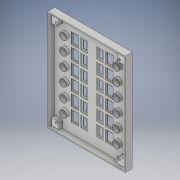
# Autodesk Inventor part: TestTapa_v2
Saved by Autodesk Inventor 2019 (Build 230136000, 136)
## iProperties
Created: 2019-05-27
Part Number: TestTapa_v2
Material: Genérico
Document SubType Name: Modeling
Designer: LuisAlonso
Density: 1 g/cm^3
Appearance: Valor por defecto
Author: LuisAlonso
Autodesk Inventor part; units mm, degrees
(part 1 of 2)
ref_plane "YZ Plane" through (0, 0, 0) normal (1, 0, 0) x (0, 1, 0)
ref_plane "XZ Plane" through (0, 0, 0) normal (0, 1, 0) x (-1, 0, 0)
ref_plane "XY Plane" through (0, 0, 0) normal (0, 0, 1) x (1, 0, 0)
sketch "Boceto1" plane through (0, 0, 0) normal (0, 0, 1) x (1, 0, 0)
  line L0 (-83, -108.2) -> (83, -108.2)
  line L1 (83, -108.2) -> (83, 108.2)
  line L2 (83, 108.2) -> (-83, 108.2)
  line L3 (-83, 108.2) -> (-83, -108.2)
  line L4 (-83, -108.2) -> (83, 108.2) construction
  line L5 (83, -108.2) -> (-83, 108.2) construction
  point P0 (0, 0)
  dimension "d0" = 166
  dimension "d1" = 216.4
  constraints: 12 end point, 2 midpoint, 2 parallel, 1 horizontal, 1 perpendicular
  measures "d0" distance of L2.end L1.end
  measures "d1" distance of L1.end L0.end
extrude "Extrusión1" add sketch "Boceto1" along normal blind 15
sketch "Boceto2" plane through (0, 0, 15) normal (0, 0, 1) x (1, 0, 0)
  line L0 (80.75, -105.95) -> (-80.75, -105.95)
  line L1 (-80.75, -105.95) -> (-80.75, 105.95)
  line L2 (80.75, 105.95) -> (-80.75, 105.95)
  line L3 (80.75, 105.95) -> (80.75, -105.95)
  line L4 (-83, 108.2) -> (83, 108.2)
  line L5 (83, 108.2) -> (83, -108.2)
  line L6 (83, -108.2) -> (-83, -108.2)
  line L7 (-83, -108.2) -> (-83, 108.2)
  point P0 (0, 0)
  constraints: 16 end point, 4 perpendicular, 2 parallel, 1 horizontal
extrude "Extrusión2" cut sketch "Boceto2" against normal blind 12 contours L0 L1 L2 L3
sketch "Boceto3" plane through (0, 0, 3) normal (0, 0, 1) x (1, 0, 0)
  line L0 (-67.5, -92.5) -> (67.5, -92.5)
  line L1 (67.5, -92.5) -> (67.5, 92.5)
  line L2 (67.5, 92.5) -> (-67.5, 92.5)
  line L3 (-67.5, 92.5) -> (-67.5, -92.5)
  line L4 (-67.5, 87.5) -> (-72.5, 87.5)
  line L5 (-62.5, 97.5) -> (-62.5, 92.5)
  line L6 (62.5, -97.5) -> (62.5, -92.5)
  line L7 (67.5, -87.5) -> (72.5, -87.5)
  line L8 (-72.5, -87.5) -> (-67.5, -87.5)
  line L9 (-62.5, -92.5) -> (-62.5, -97.5)
  line L10 (-72.5, 87.5) -> (-77.5, 87.5)
  line L11 (-77.5, 87.5) -> (-77.5, 102.5)
  line L12 (-77.5, 102.5) -> (-62.5, 102.5)
  line L13 (-62.5, 102.5) -> (-62.5, 97.5)
  line L14 (77.5, 87.5) -> (77.5, 102.5)
  line L15 (77.5, 102.5) -> (62.5, 102.5)
  line L16 (67.5, -87.5) -> (77.5, -87.5)
  line L17 (62.5, -92.5) -> (62.5, -102.5)
  line L18 (62.5, -102.5) -> (77.5, -102.5)
  line L19 (77.5, -102.5) -> (77.5, -87.5)
  line L20 (-67.5, -87.5) -> (-77.5, -87.5)
  line L21 (-77.5, -87.5) -> (-77.5, -102.5)
  line L22 (-77.5, -102.5) -> (-62.5, -102.5)
  line L23 (-62.5, -102.5) -> (-62.5, -97.5)
  line L24 (67.5, 87.5) -> (77.5, 87.5)
  line L25 (62.5, 102.5) -> (62.5, 92.5)
  arc A0 (-62.5, -92.5) -> (-67.5, -87.5) centre (-67.5, -92.5) ccw
  arc A1 (-67.5, 87.5) -> (-62.5, 92.5) centre (-67.5, 92.5) ccw
  arc A2 (62.5, 92.5) -> (67.5, 87.5) centre (67.5, 92.5) ccw
  arc A3 (67.5, -87.5) -> (62.5, -92.5) centre (67.5, -92.5) ccw
  point P0 (0, 0)
  dimension "d12" = 135
  dimension "d13" = 185
  dimension "d56" = 5
  dimension "d57" = 15
  dimension "d58" = 15
  constraints: 52 end point, 10 perpendicular, 8 point on circle, 6 point on line, 4 centre point, 4 coincident, 4 horizontal, 3 vertical, 2 midpoint, 1 collinear
  measures "d12" distance of L0.start L0.end
  measures "d13" distance of L0.end L1.end
  measures "d56" distance of L4.end L10.end
  measures "d57" distance of L10.end L11.end
  measures "d58" distance of L11.end L12.end
extrude "Extrusión3" add sketch "Boceto3" along normal blind 9 contours L3 A0 L0 | L0 L9 L23 L22 L21 L20 L8 L3 | A3 L1 L0 | L0 L1 L7 L16 L19 L18 L17 L6 | L4 L10 L11 L12 L13 L5 L2 L3 | L3 L2 A1 | A2 L2 L1 | L1 L2 L25 L15 L14 L24
sketch "Boceto4" plane through (0, 0, 0) normal (0, 0, -1) x (-1, 0, 0)
  line L0 (80.75, -105.95) -> (80.75, 105.95) projected
  line L1 (-80.75, -105.95) -> (80.75, -105.95) projected
  line L2 (-80.75, 105.95) -> (-80.75, -105.95) projected
  line L3 (80.75, 105.95) -> (-80.75, 105.95) projected
  line L4 (-67.5, -92.5) -> (-67.5, 92.5) projected
  line L5 (67.5, 92.5) -> (67.5, -92.5) projected
  line L6 (-67.5, 92.5) -> (67.5, 92.5) projected
  line L7 (67.5, -92.5) -> (-67.5, -92.5) projected
  circle A0 centre (-67.5, 92.5) radius 4.75
  circle A1 centre (67.5, 92.5) radius 4.75
  circle A2 centre (67.5, -92.5) radius 4.75
  circle A3 centre (-67.5, -92.5) radius 4.75
  point P0 (0, 0)
  dimension "d24" = 9.5
  dimension "d25" = 9.5
  dimension "d26" = 9.5
  dimension "d27" = 9.5
  constraints: 4 centre point, 4 coincident
  measures "d24" diameter of A0
  measures "d25" diameter of A1
  measures "d26" diameter of A2
  measures "d27" diameter of A3
extrude "Extrusión4" cut sketch "Boceto4" against normal blind 4.5 contours L7 A3 L4 | L4 A3 L7 | A0 L6 L4 | L4 L6 A0 | A2 L5 L7 | L7 L5 A2 | A1 L5 L6 | L6 L5 A1
sketch "Boceto7" plane through (-67.5, 92.5, 4.5) normal (0, 0, -1) x (-1, 0, 0)
  arc A0 (-0.8744, -2.2886) -> (-2.2886, -0.8744) centre (0, 0) ccw
  line L0 (0, 0) -> (4.75, 0) construction
  line L1 (-2.2886, -0.8744) -> (-3.9906, -2.5764)
  line L2 (-0.8744, -2.2886) -> (-2.5764, -3.9906)
  arc A1 (-3.9906, -2.5764) -> (-2.5764, -3.9906) centre (0, 0) ccw
  arc A2 (-132.7114, -0.8744) -> (-134.1256, -2.2886) centre (-135, 0) ccw
  line L3 (-134.1256, -2.2886) -> (-132.4236, -3.9906)
  line L4 (-132.7114, -0.8744) -> (-131.0094, -2.5764)
  arc A3 (-132.4236, -3.9906) -> (-131.0094, -2.5764) centre (-135, 0) ccw
  arc A4 (-134.1256, -182.7114) -> (-132.7114, -184.1256) centre (-135, -185) ccw
  line L5 (-132.7114, -184.1256) -> (-131.0094, -182.4236)
  line L6 (-134.1256, -182.7114) -> (-132.4236, -181.0094)
  arc A5 (-131.0094, -182.4236) -> (-132.4236, -181.0094) centre (-135, -185) ccw
  arc A6 (-2.2886, -184.1256) -> (-0.8744, -182.7114) centre (0, -185) ccw
  line L7 (-0.8744, -182.7114) -> (-2.5764, -181.0094)
  line L8 (-2.2886, -184.1256) -> (-3.9906, -182.4236)
  arc A7 (-2.5764, -181.0094) -> (-3.9906, -182.4236) centre (0, -185) ccw
  point P0 (-67.5, -92.5)
  constraints: 18 end point, 16 point on circle, 8 centre point, 1 horizontal
extrude "Extrusión7" cut sketch "Boceto7" against normal blind 10
sketch "Boceto8" plane through (0, 0, 3) normal (0, 0, 1) x (1, 0, 0)
  line L0 (80.75, -105.95) -> (-80.75, -105.95) projected
  line L1 (-62.5, -105.95) -> (-57.5, -105.95)
  line L2 (-57.5, -100.95) -> (57.5161, -100.95)
  line L3 (67.5, -87.5) -> (77.5, -87.5) projected
  line L4 (57.5161, -92.5) -> (57.5161, -100.95)
  line L5 (-57.5, -100.95) -> (-57.5, -92.5)
  line L6 (-67.5, -82.5) -> (-75.75, -82.5)
  line L7 (-77.5, 87.5) -> (-67.5, 87.5) projected
  line L8 (-62.5, 92.5) -> (-62.5, 102.5) projected
  line L9 (-80.75, 105.95) -> (80.75, 105.95) projected
  line L10 (-75.75, 82.5) -> (-67.5, 82.5)
  line L11 (-57.5, 92.5) -> (-57.5, 100.95)
  line L12 (-75.75, -82.5) -> (-75.75, 82.5)
  line L13 (-57.5, 100.95) -> (57.5161, 100.95)
  line L14 (57.5161, 100.95) -> (57.5161, 91.9319)
  line L15 (67.5, 82.5) -> (75.75, 82.5)
  line L16 (75.75, 82.5) -> (75.75, -82.5161)
  arc A0 (65.2114, -91.6256) -> (66.6256, -90.2114) centre (67.5, -92.5) ccw projected
  line L17 (67.5, -82.5161) -> (75.75, -82.5161)
  arc A1 (-66.6256, -90.2114) -> (-65.2114, -91.6256) centre (-67.5, -92.5) ccw projected
  arc A2 (-57.5, -92.5) -> (-67.5, -82.5) centre (-67.5, -92.5) ccw
  arc A3 (-65.2114, 91.6256) -> (-66.6256, 90.2114) centre (-67.5, 92.5) ccw projected
  arc A4 (-67.5, 82.5) -> (-57.5, 92.5) centre (-67.5, 92.5) ccw
  arc A5 (67.5, -82.5161) -> (57.5161, -92.5) centre (67.5, -92.5) ccw
  arc A6 (66.6256, 90.2114) -> (65.2114, 91.6256) centre (67.5, 92.5) ccw projected
  arc A7 (57.5, 92.5) -> (67.5, 82.5) centre (67.5, 92.5) ccw
  point P0 (0, 0)
  constraints: 26 end point, 9 point on circle, 4 centre point, 4 coincident, 4 horizontal, 4 perpendicular, 2 point on line, 2 vertical
sketch "Boceto9" plane through (0, 0, 3) normal (0, 0, 1) x (1, 0, 0)
  line L0 (0, 100.8776) -> (0, -101.1224)
  line L1 (0, 100.8776) -> (0, 72.0206)
  line L2 (0, 72.0206) -> (0, 43.1636)
  line L3 (0, 43.1636) -> (0, 14.3066)
  line L4 (0, 14.3066) -> (0, -14.5504)
  line L5 (0, -14.5504) -> (0, -43.4074)
  line L6 (0, -43.4074) -> (0, -72.2644)
  line L7 (0, -72.2644) -> (0, -101.1214)
  line L8 (0, 72.0206) -> (10, 72.0206)
  line L9 (10, 72.0206) -> (24, 72.0206)
  line L10 (24, 72.0206) -> (29, 72.0206)
  line L11 (29, 72.0206) -> (45, 72.0206)
  line L12 (45, 72.0206) -> (50, 72.0206)
  line L13 (50, 72.0206) -> (56.75, 72.0206)
  circle A0 centre (56.75, 72.0206) radius 6.75
  line L14 (30.5, 62.1456) -> (30.5, 81.8956)
  line L15 (30.5, 81.8956) -> (43.5, 81.8956)
  line L16 (43.5, 81.8956) -> (43.5, 62.1456)
  line L17 (43.5, 62.1456) -> (30.5, 62.1456)
  line L18 (30.5, 62.1456) -> (43.5, 81.8956) construction
  line L19 (30.5, 81.8956) -> (43.5, 62.1456) construction
  line L20 (13, 63.5206) -> (13, 80.5206)
  line L21 (13, 80.5206) -> (21, 80.5206)
  line L22 (21, 80.5206) -> (21, 63.5206)
  line L23 (21, 63.5206) -> (13, 63.5206)
  line L24 (13, 63.5206) -> (21, 80.5206) construction
  line L25 (13, 80.5206) -> (21, 63.5206) construction
  line L26 (0, 72.0206) -> (-10, 72.0206)
  line L27 (-10, 72.0206) -> (-24, 72.0206)
  line L28 (-24, 72.0206) -> (-29, 72.0206)
  line L29 (-29, 72.0206) -> (-45, 72.0206)
  line L30 (-45, 72.0206) -> (-50, 72.0206)
  line L31 (-50, 72.0206) -> (-56.75, 72.0206)
  circle A1 centre (-56.75, 72.0206) radius 6.75
  line L32 (-30.5, 62.1456) -> (-30.5, 81.8956)
  line L33 (-30.5, 81.8956) -> (-43.5, 81.8956)
  line L34 (-43.5, 81.8956) -> (-43.5, 62.1456)
  line L35 (-43.5, 62.1456) -> (-30.5, 62.1456)
  line L36 (-30.5, 62.1456) -> (-43.5, 81.8956) construction
  line L37 (-30.5, 81.8956) -> (-43.5, 62.1456) construction
  line L38 (-13, 63.5206) -> (-13, 80.5206)
  line L39 (-13, 80.5206) -> (-21, 80.5206)
  line L40 (-21, 80.5206) -> (-21, 63.5206)
  line L41 (-21, 63.5206) -> (-13, 63.5206)
  line L42 (-13, 63.5206) -> (-21, 80.5206) construction
  line L43 (-13, 80.5206) -> (-21, 63.5206) construction
  line L44 (0, 43.1636) -> (10, 43.1636)
  line L45 (10, 43.1636) -> (24, 43.1636)
  line L46 (24, 43.1636) -> (29, 43.1636)
  line L47 (29, 43.1636) -> (45, 43.1636)
  line L48 (45, 43.1636) -> (50, 43.1636)
  line L49 (50, 43.1636) -> (56.75, 43.1636)
  circle A2 centre (56.75, 43.1636) radius 6.75
  line L50 (30.5, 33.2886) -> (30.5, 53.0386)
  line L51 (30.5, 53.0386) -> (43.5, 53.0386)
  line L52 (43.5, 53.0386) -> (43.5, 33.2886)
  line L53 (43.5, 33.2886) -> (30.5, 33.2886)
  line L54 (30.5, 33.2886) -> (43.5, 53.0386) construction
  line L55 (30.5, 53.0386) -> (43.5, 33.2886) construction
  line L56 (13, 34.6636) -> (13, 51.6636)
  line L57 (13, 51.6636) -> (21, 51.6636)
  line L58 (21, 51.6636) -> (21, 34.6636)
  line L59 (21, 34.6636) -> (13, 34.6636)
  line L60 (13, 34.6636) -> (21, 51.6636) construction
  line L61 (13, 51.6636) -> (21, 34.6636) construction
  line L62 (-30.5, 33.2886) -> (-30.5, 53.0386)
  line L63 (-43.5, 33.2886) -> (-30.5, 33.2886)
  line L64 (-30.5, 33.2886) -> (-43.5, 53.0386) construction
  line L65 (-30.5, 53.0386) -> (-43.5, 33.2886) construction
  line L66 (-30.5, 53.0386) -> (-43.5, 53.0386)
  line L67 (-29, 43.1636) -> (-45, 43.1636)
  line L68 (-43.5, 53.0386) -> (-43.5, 33.2886)
  line L69 (-45, 43.1636) -> (-50, 43.1636)
  line L70 (-50, 43.1636) -> (-56.75, 43.1636)
  circle A3 centre (-56.75, 43.1636) radius 6.75
  line L71 (-21, 34.6636) -> (-13, 34.6636)
  line L72 (0, 43.1636) -> (-10, 43.1636)
  line L73 (-10, 43.1636) -> (-24, 43.1636)
  line L74 (-24, 43.1636) -> (-29, 43.1636)
  line L75 (-13, 34.6636) -> (-13, 51.6636)
  line L76 (-21, 51.6636) -> (-21, 34.6636)
  line L77 (-13, 51.6636) -> (-21, 51.6636)
  line L78 (-13, 34.6636) -> (-21, 51.6636) construction
  line L79 (-13, 51.6636) -> (-21, 34.6636) construction
  line L80 (0, 14.3066) -> (10, 14.3066)
  line L81 (10, 14.3066) -> (24, 14.3066)
  line L82 (24, 14.3066) -> (29, 14.3066)
  line L83 (29, 14.3066) -> (45, 14.3066)
  line L84 (45, 14.3066) -> (50, 14.3066)
  line L85 (50, 14.3066) -> (56.75, 14.3066)
  circle A4 centre (56.75, 14.3066) radius 6.75
  line L86 (30.5, 4.4316) -> (30.5, 24.1816)
  line L87 (30.5, 24.1816) -> (43.5, 24.1816)
  line L88 (43.5, 24.1816) -> (43.5, 4.4316)
  line L89 (43.5, 4.4316) -> (30.5, 4.4316)
  line L90 (30.5, 4.4316) -> (43.5, 24.1816) construction
  line L91 (30.5, 24.1816) -> (43.5, 4.4316) construction
  line L92 (13, 5.8066) -> (13, 22.8066)
  line L93 (13, 22.8066) -> (21, 22.8066)
  line L94 (21, 22.8066) -> (21, 5.8066)
  line L95 (21, 5.8066) -> (13, 5.8066)
  line L96 (13, 5.8066) -> (21, 22.8066) construction
  line L97 (13, 22.8066) -> (21, 5.8066) construction
  line L98 (-30.5, 4.4316) -> (-30.5, 24.1816)
  line L99 (-43.5, 4.4316) -> (-30.5, 4.4316)
  line L100 (-30.5, 4.4316) -> (-43.5, 24.1816) construction
  line L101 (-30.5, 24.1816) -> (-43.5, 4.4316) construction
  line L102 (-30.5, 24.1816) -> (-43.5, 24.1816)
  line L103 (-29, 14.3066) -> (-45, 14.3066)
  line L104 (-43.5, 24.1816) -> (-43.5, 4.4316)
  line L105 (-45, 14.3066) -> (-50, 14.3066)
  line L106 (-50, 14.3066) -> (-56.75, 14.3066)
  circle A5 centre (-56.75, 14.3066) radius 6.75
  line L107 (-21, 5.8066) -> (-13, 5.8066)
  line L108 (0, 14.3066) -> (-10, 14.3066)
  line L109 (-10, 14.3066) -> (-24, 14.3066)
  line L110 (-24, 14.3066) -> (-29, 14.3066)
  line L111 (-13, 5.8066) -> (-13, 22.8066)
  line L112 (-21, 22.8066) -> (-21, 5.8066)
  line L113 (-13, 22.8066) -> (-21, 22.8066)
  line L114 (-13, 5.8066) -> (-21, 22.8066) construction
  line L115 (-13, 22.8066) -> (-21, 5.8066) construction
  line L116 (0, -14.5504) -> (10, -14.5504)
  line L117 (10, -14.5504) -> (24, -14.5504)
  line L118 (24, -14.5504) -> (29, -14.5504)
  line L119 (29, -14.5504) -> (45, -14.5504)
  line L120 (45, -14.5504) -> (50, -14.5504)
  line L121 (50, -14.5504) -> (56.75, -14.5504)
  circle A6 centre (56.75, -14.5504) radius 6.75
  line L122 (30.5, -24.4254) -> (30.5, -4.6754)
  line L123 (30.5, -4.6754) -> (43.5, -4.6754)
  line L124 (43.5, -4.6754) -> (43.5, -24.4254)
  line L125 (43.5, -24.4254) -> (30.5, -24.4254)
  line L126 (30.5, -24.4254) -> (43.5, -4.6754) construction
  line L127 (30.5, -4.6754) -> (43.5, -24.4254) construction
  line L128 (13, -23.0504) -> (13, -6.0504)
  line L129 (13, -6.0504) -> (21, -6.0504)
  line L130 (21, -6.0504) -> (21, -23.0504)
  line L131 (21, -23.0504) -> (13, -23.0504)
  line L132 (13, -23.0504) -> (21, -6.0504) construction
  line L133 (13, -6.0504) -> (21, -23.0504) construction
  line L134 (-30.5, -24.4254) -> (-30.5, -4.6754)
  line L135 (-43.5, -24.4254) -> (-30.5, -24.4254)
  line L136 (-30.5, -24.4254) -> (-43.5, -4.6754) construction
  line L137 (-30.5, -4.6754) -> (-43.5, -24.4254) construction
  line L138 (-30.5, -4.6754) -> (-43.5, -4.6754)
  line L139 (-29, -14.5504) -> (-45, -14.5504)
  line L140 (-43.5, -4.6754) -> (-43.5, -24.4254)
  line L141 (-45, -14.5504) -> (-50, -14.5504)
  line L142 (-50, -14.5504) -> (-56.75, -14.5504)
  circle A7 centre (-56.75, -14.5504) radius 6.75
  line L143 (-21, -23.0504) -> (-13, -23.0504)
  line L144 (0, -14.5504) -> (-10, -14.5504)
  line L145 (-10, -14.5504) -> (-24, -14.5504)
  line L146 (-24, -14.5504) -> (-29, -14.5504)
  line L147 (-13, -23.0504) -> (-13, -6.0504)
  line L148 (-21, -6.0504) -> (-21, -23.0504)
  line L149 (-13, -6.0504) -> (-21, -6.0504)
  line L150 (-13, -23.0504) -> (-21, -6.0504) construction
  line L151 (-13, -6.0504) -> (-21, -23.0504) construction
  line L152 (0, -43.4074) -> (10, -43.4074)
  line L153 (10, -43.4074) -> (24, -43.4074)
  line L154 (24, -43.4074) -> (29, -43.4074)
  line L155 (29, -43.4074) -> (45, -43.4074)
  line L156 (45, -43.4074) -> (50, -43.4074)
  line L157 (50, -43.4074) -> (56.75, -43.4074)
  circle A8 centre (56.75, -43.4074) radius 6.75
  line L158 (30.5, -53.2824) -> (30.5, -33.5324)
  line L159 (30.5, -33.5324) -> (43.5, -33.5324)
  line L160 (43.5, -33.5324) -> (43.5, -53.2824)
  line L161 (43.5, -53.2824) -> (30.5, -53.2824)
  line L162 (30.5, -53.2824) -> (43.5, -33.5324) construction
  line L163 (30.5, -33.5324) -> (43.5, -53.2824) construction
  line L164 (13, -51.9074) -> (13, -34.9074)
  line L165 (13, -34.9074) -> (21, -34.9074)
  line L166 (21, -34.9074) -> (21, -51.9074)
  line L167 (21, -51.9074) -> (13, -51.9074)
  line L168 (13, -51.9074) -> (21, -34.9074) construction
  line L169 (13, -34.9074) -> (21, -51.9074) construction
  line L170 (-30.5, -53.2824) -> (-30.5, -33.5324)
  line L171 (-43.5, -53.2824) -> (-30.5, -53.2824)
  line L172 (-30.5, -53.2824) -> (-43.5, -33.5324) construction
  line L173 (-30.5, -33.5324) -> (-43.5, -53.2824) construction
  line L174 (-30.5, -33.5324) -> (-43.5, -33.5324)
  line L175 (-29, -43.4074) -> (-45, -43.4074)
  line L176 (-43.5, -33.5324) -> (-43.5, -53.2824)
  line L177 (-45, -43.4074) -> (-50, -43.4074)
  line L178 (-50, -43.4074) -> (-56.75, -43.4074)
  circle A9 centre (-56.75, -43.4074) radius 6.75
  line L179 (-21, -51.9074) -> (-13, -51.9074)
  line L180 (0, -43.4074) -> (-10, -43.4074)
  line L181 (-10, -43.4074) -> (-24, -43.4074)
  line L182 (-24, -43.4074) -> (-29, -43.4074)
  line L183 (-13, -51.9074) -> (-13, -34.9074)
  line L184 (-21, -34.9074) -> (-21, -51.9074)
  line L185 (-13, -34.9074) -> (-21, -34.9074)
  line L186 (-13, -51.9074) -> (-21, -34.9074) construction
  line L187 (-13, -34.9074) -> (-21, -51.9074) construction
  line L188 (0, -72.2644) -> (10, -72.2644)
  line L189 (10, -72.2644) -> (24, -72.2644)
  line L190 (24, -72.2644) -> (29, -72.2644)
  line L191 (29, -72.2644) -> (45, -72.2644)
  line L192 (45, -72.2644) -> (50, -72.2644)
  line L193 (50, -72.2644) -> (56.75, -72.2644)
  circle A10 centre (56.75, -72.2644) radius 6.75
  line L194 (30.5, -82.1394) -> (30.5, -62.3894)
  line L195 (30.5, -62.3894) -> (43.5, -62.3894)
  line L196 (43.5, -62.3894) -> (43.5, -82.1394)
  line L197 (43.5, -82.1394) -> (30.5, -82.1394)
  line L198 (30.5, -82.1394) -> (43.5, -62.3894) construction
  line L199 (30.5, -62.3894) -> (43.5, -82.1394) construction
  line L200 (13, -80.7644) -> (13, -63.7644)
  line L201 (13, -63.7644) -> (21, -63.7644)
  line L202 (21, -63.7644) -> (21, -80.7644)
  line L203 (21, -80.7644) -> (13, -80.7644)
  line L204 (13, -80.7644) -> (21, -63.7644) construction
  line L205 (13, -63.7644) -> (21, -80.7644) construction
  line L206 (-30.5, -82.1394) -> (-30.5, -62.3894)
  line L207 (-43.5, -82.1394) -> (-30.5, -82.1394)
  line L208 (-30.5, -82.1394) -> (-43.5, -62.3894) construction
  line L209 (-30.5, -62.3894) -> (-43.5, -82.1394) construction
  line L210 (-30.5, -62.3894) -> (-43.5, -62.3894)
  line L211 (-29, -72.2644) -> (-45, -72.2644)
  line L212 (-43.5, -62.3894) -> (-43.5, -82.1394)
  line L213 (-45, -72.2644) -> (-50, -72.2644)
  line L214 (-50, -72.2644) -> (-56.75, -72.2644)
  circle A11 centre (-56.75, -72.2644) radius 6.75
  line L215 (-21, -80.7644) -> (-13, -80.7644)
  line L216 (0, -72.2644) -> (-10, -72.2644)
  line L217 (-10, -72.2644) -> (-24, -72.2644)
  line L218 (-24, -72.2644) -> (-29, -72.2644)
  line L219 (-13, -80.7644) -> (-13, -63.7644)
  line L220 (-21, -63.7644) -> (-21, -80.7644)
  line L221 (-13, -63.7644) -> (-21, -63.7644)
  line L222 (-13, -80.7644) -> (-21, -63.7644) construction
  line L223 (-13, -63.7644) -> (-21, -80.7644) construction
  point P0 (0, 0)
  point P1 (37, 72.0206)
  point P2 (17, 72.0206)
  point P3 (-37, 72.0206)
  point P4 (-17, 72.0206)
  point P5 (37, 43.1636)
  point P6 (17, 43.1636)
  point P7 (-37, 43.1636)
  point P8 (-17, 43.1636)
  point P9 (37, 14.3066)
  point P10 (17, 14.3066)
  point P11 (-37, 14.3066)
  point P12 (-17, 14.3066)
  point P13 (37, -14.5504)
  point P14 (17, -14.5504)
  point P15 (-37, -14.5504)
  point P16 (-17, -14.5504)
  point P17 (37, -43.4074)
  point P18 (17, -43.4074)
  point P19 (-37, -43.4074)
  point P20 (-17, -43.4074)
  point P21 (37, -72.2644)
  point P22 (17, -72.2644)
  point P23 (-37, -72.2644)
  point P24 (-17, -72.2644)
  dimension "d119" = 202
  dimension "d120" = 28.857
  dimension "d121" = 28.857
  dimension "d122" = 28.857
  dimension "d123" = 28.857
  dimension "d124" = 28.857
  dimension "d125" = 28.857
  dimension "d126" = 28.857
  dimension "d128" = 10
  dimension "d130" = 14
  dimension "d131" = 5
  dimension "d132" = 16
  dimension "d133" = 5
  dimension "d134" = 6.75
  dimension "d135" = 13.5
  dimension "d136" = 19.75
  dimension "d137" = 13
  dimension "d138" = 17
  dimension "d139" = 8
  dimension "d140" = 10
  dimension "d141" = 14
  dimension "d142" = 5
  dimension "d143" = 16
  dimension "d144" = 5
  dimension "d145" = 6.75
  dimension "d146" = 13.5
  dimension "d147" = 19.75
  dimension "d148" = 13
  dimension "d149" = 17
  dimension "d150" = 8
  dimension "d151" = 10
  dimension "d152" = 14
  dimension "d153" = 5
  dimension "d154" = 16
  dimension "d155" = 5
  dimension "d156" = 6.75
  dimension "d157" = 13.5
  dimension "d158" = 19.75
  dimension "d159" = 13
  dimension "d160" = 17
  dimension "d161" = 8
  dimension "d162" = 10
  dimension "d163" = 14
  dimension "d164" = 5
  dimension "d165" = 16
  dimension "d166" = 5
  dimension "d167" = 6.75
  dimension "d168" = 13.5
  dimension "d169" = 19.75
  dimension "d170" = 13
  dimension "d171" = 17
  dimension "d172" = 8
  dimension "d173" = 10
  dimension "d174" = 14
  dimension "d175" = 5
  dimension "d176" = 16
  dimension "d177" = 5
  dimension "d178" = 6.75
  dimension "d179" = 13.5
  dimension "d180" = 19.75
  dimension "d181" = 13
  dimension "d182" = 17
  dimension "d183" = 8
  dimension "d184" = 10
  constraints: 446 end point, 60 midpoint, 48 point on line, 24 parallel, 24 perpendicular, 17 symmetric about line, 12 centre point, 12 coincident, 12 horizontal, 11 other
  measures "d119" distance of L1.start point (0, -101.122)
  measures "d120" distance of L1.start L1.end
  measures "d121" distance of L1.end L2.end
  measures "d122" distance of L2.end L3.end
  measures "d123" distance of L3.end L4.end
  measures "d124" distance of L4.end L5.end
  measures "d125" distance of L5.end L6.end
  measures "d126" distance of L6.end L7.end
  measures "d128" distance of L1.end L8.end
  measures "d130" distance of L8.end L9.end
  measures "d131" distance of L9.end L10.end
  measures "d132" distance of L10.end L11.end
  measures "d133" distance of L11.end L12.end
  measures "d134" distance of L12.end L13.end
  measures "d135" diameter of A0
  measures "d136" distance of L14.start L14.end
  measures "d137" distance of L14.end L15.end
  measures "d138" distance of L20.start L20.end
  measures "d139" distance of L20.end L21.end
  measures "d140" distance of L44.start L44.end
  measures "d141" distance of L44.end L46.start
  measures "d142" distance of L46.start L47.start
  measures "d143" distance of L47.start L47.end
  measures "d144" distance of L47.end L48.end
  measures "d145" distance of L48.end L49.end
  measures "d146" diameter of A2
  measures "d147" distance of L54.start L55.start
  measures "d148" distance of L55.start L52.start
  measures "d149" distance of L56.start L56.end
  measures "d150" distance of L56.end L58.start
  measures "d151" distance of L80.start L80.end
  measures "d152" distance of L80.end L82.start
  measures "d153" distance of L82.start L83.start
  measures "d154" distance of L83.start L83.end
  measures "d155" distance of L83.end L84.end
  measures "d156" distance of L84.end L85.end
  measures "d157" diameter of A4
  measures "d158" distance of L90.start L91.start
  measures "d159" distance of L91.start L88.start
  measures "d160" distance of L92.start L92.end
  measures "d161" distance of L92.end L94.start
  measures "d162" distance of L116.start L116.end
  measures "d163" distance of L116.end L118.start
  measures "d164" distance of L118.start L119.start
  measures "d165" distance of L119.start L119.end
  measures "d166" distance of L119.end L120.end
  measures "d167" distance of L120.end L121.end
  measures "d168" diameter of A6
  measures "d169" distance of L126.start L127.start
  measures "d170" distance of L127.start L124.start
  measures "d171" distance of L128.start L128.end
  measures "d172" distance of L128.end L130.start
  measures "d173" distance of L152.start L152.end
  measures "d174" distance of L152.end L154.start
  measures "d175" distance of L154.start L155.start
  measures "d176" distance of L155.start L155.end
  measures "d177" distance of L155.end L156.end
  measures "d178" distance of L156.end L157.end
  measures "d179" diameter of A8
  measures "d180" distance of L162.start L163.start
  measures "d181" distance of L163.start L160.start
  measures "d182" distance of L164.start L164.end
  measures "d183" distance of L164.end L166.start
  measures "d184" distance of L188.start L188.end
extrude "Extrusión9" cut sketch "Boceto9" against normal blind 10
sketch "Boceto10" plane through (0, 0, 3) normal (0, 0, 1) x (1, 0, 0)
  circle A0 centre (-56.75, -72.2644) radius 6.75 projected
  circle A1 centre (-56.75, -72.2644) radius 8
  circle A2 centre (-56.75, -43.4074) radius 6.75 projected
  circle A3 centre (-56.75, -43.4074) radius 8
  circle A4 centre (-56.75, -14.5504) radius 8
  circle A5 centre (-56.75, 14.3066) radius 8
  circle A6 centre (-56.75, 43.1636) radius 8
  circle A7 centre (-56.75, 72.0206) radius 8
  circle A8 centre (56.75, -72.2644) radius 6.75 projected
  circle A9 centre (56.75, -72.2644) radius 8
  circle A10 centre (56.75, -43.4074) radius 8
  circle A11 centre (56.75, -14.5504) radius 8
  circle A12 centre (56.75, 14.3066) radius 8
  circle A13 centre (56.75, 43.1636) radius 8
  circle A14 centre (56.75, 72.0206) radius 8
  point P0 (0, 0)
  dimension "d197" = 16
  dimension "d198" = 16
  dimension "d199" = 16
  dimension "d200" = 16
  dimension "d201" = 16
  dimension "d202" = 16
  dimension "d203" = 16
  dimension "d204" = 16
  dimension "d205" = 16
  dimension "d206" = 16
  dimension "d207" = 16
  dimension "d208" = 16
  constraints: 12 centre point, 1 coincident
  measures "d197" diameter of A1
  measures "d198" diameter of A3
  measures "d199" diameter of A4
  measures "d200" diameter of A5
  measures "d201" diameter of A6
  measures "d202" diameter of A7
  measures "d203" diameter of A9
  measures "d204" diameter of A10
  measures "d205" diameter of A11
  measures "d206" diameter of A12
  measures "d207" diameter of A13
  measures "d208" diameter of A14
extrude "Extrusión10" add sketch "Boceto10" along normal blind 5.5
sketch "Boceto11" plane through (-56.75, -14.5504, 8.5) normal (0, 0, 1) x (1, 0, 0)
  circle A0 centre (0, 0) radius 6.75
  circle A1 centre (0, -28.857) radius 6.75 projected
  line L0 (0, 0) -> (0, -28.857)
  circle A2 centre (0, 28.857) radius 6.75
  line L1 (0, 28.857) -> (0, 0)
  circle A3 centre (0, 57.714) radius 6.75
  line L2 (0, 57.714) -> (0, 28.857)
  circle A4 centre (0, 86.571) radius 6.75
  line L3 (0, 86.571) -> (0, 57.714)
  circle A5 centre (113.5, -28.857) radius 6.75 projected
  line L4 (0, -28.857) -> (113.5, -28.857)
  circle A6 centre (113.5, -28.857) radius 6.75
  circle A7 centre (113.5, -57.714) radius 6.75 projected
  line L5 (113.5, -28.857) -> (113.5, -57.714)
  circle A8 centre (113.5, 0) radius 6.75
  line L6 (113.5, 0) -> (113.5, -28.857)
  circle A9 centre (113.5, 28.857) radius 6.75
  line L7 (113.5, 28.857) -> (113.5, 0)
  circle A10 centre (113.5, 57.714) radius 6.75
  line L8 (113.5, 57.714) -> (113.5, 28.857)
  circle A11 centre (113.5, 86.571) radius 6.75
  line L9 (113.5, 86.571) -> (113.5, 57.714)
  point P0 (56.75, 14.5504)
  dimension "d211" = 13.5
  dimension "d212" = 13.5
  dimension "d213" = 13.5
  dimension "d214" = 13.5
  constraints: 20 end point, 9 centre point, 9 vertical, 1 coincident, 1 concentric, 1 horizontal
  measures "d211" diameter of A0
  measures "d212" diameter of A2
  measures "d213" diameter of A3
  measures "d214" diameter of A4
extrude "Extrusión11" cut sketch "Boceto11" against normal blind 15 contours A0 L0 L1 | A11 | A10 L9 L8 | L8 L9 A10 | A9 L8 L7 | L7 L8 A9 | A8 L7 L6 | L6 L7 A8 | A5 L6 L4 | L4 L5 A5 | A4 | A3 L3 L2 | L2 L3 A3 | A2 L2 L1 | L1 L2 A2 | L1 L0 A0 | A5 L5 L6
sketch "Boceto12" plane through (0, 0, 3) normal (0, 0, 1) x (1, 0, 0)
  circle A0 centre (-56.75, -72.2644) radius 6.75 projected
  line L0 (-56.75, -72.2644) -> (-37.0001, -72.2644)
  circle A1 centre (-56.75, -43.4074) radius 6.75 projected
  line L1 (-56.75, -72.2644) -> (-56.75, -43.4074)
  line L2 (-56.75, -43.4074) -> (-37.0001, -43.4074)
  line L3 (-29.0001, -84.1314) -> (-29.0001, -60.3974)
  line L4 (-29.0001, -60.3974) -> (-45.0001, -60.3974)
  line L5 (-45.0001, -60.3974) -> (-45.0001, -84.1314)
  line L6 (-45.0001, -84.1314) -> (-29.0001, -84.1314)
  line L7 (-29.0001, -84.1314) -> (-45.0001, -60.3974) construction
  line L8 (-29.0001, -60.3974) -> (-45.0001, -84.1314) construction
  line L9 (-17.0001, -72.2644) -> (-37.0001, -72.2644)
  line L10 (-24.0001, -60.7644) -> (-24.0001, -83.7644)
  line L11 (-24.0001, -83.7644) -> (-10.0001, -83.7644)
  line L12 (-10.0001, -83.7644) -> (-10.0001, -60.7644)
  line L13 (-10.0001, -60.7644) -> (-24.0001, -60.7644)
  line L14 (-24.0001, -60.7644) -> (-10.0001, -83.7644) construction
  line L15 (-24.0001, -83.7644) -> (-10.0001, -60.7644) construction
  line L16 (0, -100.98) -> (0, -43.4074)
  line L17 (29.0001, -84.1314) -> (29.0001, -60.3974)
  line L18 (29.0001, -60.3974) -> (45.0001, -60.3974)
  line L19 (45.0001, -60.3974) -> (45.0001, -84.1314)
  line L20 (45.0001, -84.1314) -> (29.0001, -84.1314)
  line L21 (29.0001, -84.1314) -> (45.0001, -60.3974) construction
  line L22 (29.0001, -60.3974) -> (45.0001, -84.1314) construction
  line L23 (24.0001, -60.7644) -> (24.0001, -83.7644)
  line L24 (24.0001, -83.7644) -> (10.0001, -83.7644)
  line L25 (10.0001, -83.7644) -> (10.0001, -60.7644)
  line L26 (10.0001, -60.7644) -> (24.0001, -60.7644)
  line L27 (24.0001, -60.7644) -> (10.0001, -83.7644) construction
  line L28 (24.0001, -83.7644) -> (10.0001, -60.7644) construction
  line L29 (-56.75, -43.4074) -> (-37.0001, -43.4074)
  line L30 (-56.75, -43.4074) -> (-56.75, -14.5504)
  line L31 (-29.0001, -55.2744) -> (-29.0001, -31.5404)
  line L32 (-29.0001, -31.5404) -> (-45.0001, -31.5404)
  line L33 (-45.0001, -31.5404) -> (-45.0001, -55.2744)
  line L34 (-45.0001, -55.2744) -> (-29.0001, -55.2744)
  line L35 (-29.0001, -55.2744) -> (-45.0001, -31.5404) construction
  line L36 (-29.0001, -31.5404) -> (-45.0001, -55.2744) construction
  line L37 (-17.0001, -43.4074) -> (-37.0001, -43.4074)
  line L38 (-24.0001, -31.9074) -> (-24.0001, -54.9074)
  line L39 (-24.0001, -54.9074) -> (-10.0001, -54.9074)
  line L40 (-10.0001, -54.9074) -> (-10.0001, -31.9074)
  line L41 (-10.0001, -31.9074) -> (-24.0001, -31.9074)
  line L42 (-24.0001, -31.9074) -> (-10.0001, -54.9074) construction
  line L43 (-24.0001, -54.9074) -> (-10.0001, -31.9074) construction
  line L44 (24.0001, -31.9074) -> (24.0001, -54.9074)
  line L45 (24.0001, -54.9074) -> (10.0001, -54.9074)
  line L46 (10.0001, -31.9074) -> (24.0001, -31.9074)
  line L47 (24.0001, -31.9074) -> (10.0001, -54.9074) construction
  line L48 (24.0001, -54.9074) -> (10.0001, -31.9074) construction
  line L49 (10.0001, -54.9074) -> (10.0001, -31.9074)
  line L50 (29.0001, -55.2744) -> (29.0001, -31.5404)
  line L51 (29.0001, -31.5404) -> (45.0001, -31.5404)
  line L52 (45.0001, -55.2744) -> (29.0001, -55.2744)
  line L53 (29.0001, -55.2744) -> (45.0001, -31.5404) construction
  line L54 (29.0001, -31.5404) -> (45.0001, -55.2744) construction
  line L55 (45.0001, -31.5404) -> (45.0001, -55.2744)
  line L56 (-56.75, -14.5504) -> (-37.0001, -14.5504)
  line L57 (-56.75, -14.5504) -> (-56.75, 14.3066)
  line L58 (-29.0001, -26.4174) -> (-29.0001, -2.6834)
  line L59 (-29.0001, -2.6834) -> (-45.0001, -2.6834)
  line L60 (-45.0001, -2.6834) -> (-45.0001, -26.4174)
  line L61 (-45.0001, -26.4174) -> (-29.0001, -26.4174)
  line L62 (-29.0001, -26.4174) -> (-45.0001, -2.6834) construction
  line L63 (-29.0001, -2.6834) -> (-45.0001, -26.4174) construction
  line L64 (-17.0001, -14.5504) -> (-37.0001, -14.5504)
  line L65 (-24.0001, -3.0504) -> (-24.0001, -26.0504)
  line L66 (-24.0001, -26.0504) -> (-10.0001, -26.0504)
  line L67 (-10.0001, -26.0504) -> (-10.0001, -3.0504)
  line L68 (-10.0001, -3.0504) -> (-24.0001, -3.0504)
  line L69 (-24.0001, -3.0504) -> (-10.0001, -26.0504) construction
  line L70 (-24.0001, -26.0504) -> (-10.0001, -3.0504) construction
  line L71 (24.0001, -3.0504) -> (24.0001, -26.0504)
  line L72 (24.0001, -26.0504) -> (10.0001, -26.0504)
  line L73 (10.0001, -3.0504) -> (24.0001, -3.0504)
  line L74 (24.0001, -3.0504) -> (10.0001, -26.0504) construction
  line L75 (24.0001, -26.0504) -> (10.0001, -3.0504) construction
  line L76 (10.0001, -26.0504) -> (10.0001, -3.0504)
  line L77 (29.0001, -26.4174) -> (29.0001, -2.6834)
  line L78 (29.0001, -2.6834) -> (45.0001, -2.6834)
  line L79 (45.0001, -26.4174) -> (29.0001, -26.4174)
  line L80 (29.0001, -26.4174) -> (45.0001, -2.6834) construction
  line L81 (29.0001, -2.6834) -> (45.0001, -26.4174) construction
  line L82 (45.0001, -2.6834) -> (45.0001, -26.4174)
  line L83 (-56.75, 14.3066) -> (-37.0001, 14.3066)
  line L84 (-56.75, 14.3066) -> (-56.75, 43.1636)
  line L85 (-29.0001, 2.4396) -> (-29.0001, 26.1736)
  line L86 (-29.0001, 26.1736) -> (-45.0001, 26.1736)
  line L87 (-45.0001, 26.1736) -> (-45.0001, 2.4396)
  line L88 (-45.0001, 2.4396) -> (-29.0001, 2.4396)
  line L89 (-29.0001, 2.4396) -> (-45.0001, 26.1736) construction
  line L90 (-29.0001, 26.1736) -> (-45.0001, 2.4396) construction
  line L91 (-17.0001, 14.3066) -> (-37.0001, 14.3066)
  line L92 (-24.0001, 25.8066) -> (-24.0001, 2.8066)
  line L93 (-24.0001, 2.8066) -> (-10.0001, 2.8066)
  line L94 (-10.0001, 2.8066) -> (-10.0001, 25.8066)
  line L95 (-10.0001, 25.8066) -> (-24.0001, 25.8066)
  line L96 (-24.0001, 25.8066) -> (-10.0001, 2.8066) construction
  line L97 (-24.0001, 2.8066) -> (-10.0001, 25.8066) construction
  line L98 (24.0001, 25.8066) -> (24.0001, 2.8066)
  line L99 (24.0001, 2.8066) -> (10.0001, 2.8066)
  line L100 (10.0001, 25.8066) -> (24.0001, 25.8066)
  line L101 (24.0001, 25.8066) -> (10.0001, 2.8066) construction
  line L102 (24.0001, 2.8066) -> (10.0001, 25.8066) construction
  line L103 (10.0001, 2.8066) -> (10.0001, 25.8066)
  line L104 (29.0001, 2.4396) -> (29.0001, 26.1736)
  line L105 (29.0001, 26.1736) -> (45.0001, 26.1736)
  line L106 (45.0001, 2.4396) -> (29.0001, 2.4396)
  line L107 (29.0001, 2.4396) -> (45.0001, 26.1736) construction
  line L108 (29.0001, 26.1736) -> (45.0001, 2.4396) construction
  line L109 (45.0001, 26.1736) -> (45.0001, 2.4396)
  line L110 (-56.75, 43.1636) -> (-37.0001, 43.1636)
  line L111 (-56.75, 43.1636) -> (-56.75, 72.0206)
  line L112 (-29.0001, 31.2966) -> (-29.0001, 55.0306)
  line L113 (-29.0001, 55.0306) -> (-45.0001, 55.0306)
  line L114 (-45.0001, 55.0306) -> (-45.0001, 31.2966)
  line L115 (-45.0001, 31.2966) -> (-29.0001, 31.2966)
  line L116 (-29.0001, 31.2966) -> (-45.0001, 55.0306) construction
  line L117 (-29.0001, 55.0306) -> (-45.0001, 31.2966) construction
  line L118 (-17.0001, 43.1636) -> (-37.0001, 43.1636)
  line L119 (-24.0001, 54.6636) -> (-24.0001, 31.6636)
  line L120 (-24.0001, 31.6636) -> (-10.0001, 31.6636)
  line L121 (-10.0001, 31.6636) -> (-10.0001, 54.6636)
  line L122 (-10.0001, 54.6636) -> (-24.0001, 54.6636)
  line L123 (-24.0001, 54.6636) -> (-10.0001, 31.6636) construction
  line L124 (-24.0001, 31.6636) -> (-10.0001, 54.6636) construction
  line L125 (24.0001, 54.6636) -> (24.0001, 31.6636)
  line L126 (24.0001, 31.6636) -> (10.0001, 31.6636)
  line L127 (10.0001, 54.6636) -> (24.0001, 54.6636)
  line L128 (24.0001, 54.6636) -> (10.0001, 31.6636) construction
  line L129 (24.0001, 31.6636) -> (10.0001, 54.6636) construction
  line L130 (10.0001, 31.6636) -> (10.0001, 54.6636)
  line L131 (29.0001, 31.2966) -> (29.0001, 55.0306)
  line L132 (29.0001, 55.0306) -> (45.0001, 55.0306)
  line L133 (45.0001, 31.2966) -> (29.0001, 31.2966)
  line L134 (29.0001, 31.2966) -> (45.0001, 55.0306) construction
  line L135 (29.0001, 55.0306) -> (45.0001, 31.2966) construction
  line L136 (45.0001, 55.0306) -> (45.0001, 31.2966)
  line L137 (-56.75, 72.0206) -> (-37.0001, 72.0206)
  line L138 (-56.75, 72.0206) -> (-56.75, 100.8776)
  line L139 (-29.0001, 60.1536) -> (-29.0001, 83.8876)
  line L140 (-29.0001, 83.8876) -> (-45.0001, 83.8876)
  line L141 (-45.0001, 83.8876) -> (-45.0001, 60.1536)
  line L142 (-45.0001, 60.1536) -> (-29.0001, 60.1536)
  line L143 (-29.0001, 60.1536) -> (-45.0001, 83.8876) construction
  line L144 (-29.0001, 83.8876) -> (-45.0001, 60.1536) construction
  line L145 (-17.0001, 72.0206) -> (-37.0001, 72.0206)
  line L146 (-24.0001, 83.5206) -> (-24.0001, 60.5206)
  line L147 (-24.0001, 60.5206) -> (-10.0001, 60.5206)
  line L148 (-10.0001, 60.5206) -> (-10.0001, 83.5206)
  line L149 (-10.0001, 83.5206) -> (-24.0001, 83.5206)
  line L150 (-24.0001, 83.5206) -> (-10.0001, 60.5206) construction
  line L151 (-24.0001, 60.5206) -> (-10.0001, 83.5206) construction
  line L152 (24.0001, 83.5206) -> (24.0001, 60.5206)
  line L153 (24.0001, 60.5206) -> (10.0001, 60.5206)
  line L154 (10.0001, 83.5206) -> (24.0001, 83.5206)
  line L155 (24.0001, 83.5206) -> (10.0001, 60.5206) construction
  line L156 (24.0001, 60.5206) -> (10.0001, 83.5206) construction
  line L157 (10.0001, 60.5206) -> (10.0001, 83.5206)
  line L158 (29.0001, 60.1536) -> (29.0001, 83.8876)
  line L159 (29.0001, 83.8876) -> (45.0001, 83.8876)
  line L160 (45.0001, 60.1536) -> (29.0001, 60.1536)
  line L161 (29.0001, 60.1536) -> (45.0001, 83.8876) construction
  line L162 (29.0001, 83.8876) -> (45.0001, 60.1536) construction
  line L163 (45.0001, 83.8876) -> (45.0001, 60.1536)
  point P0 (0, 0)
  point P1 (37.0001, -72.2644)
  point P2 (17.0001, -72.2644)
  point P3 (37.0001, -72.2644)
  point P4 (17.0001, -43.4074)
  point P5 (37.0001, -43.4074)
  point P6 (37.0001, -43.4074)
  point P7 (17.0001, -14.5504)
  point P8 (37.0001, -14.5504)
  point P9 (37.0001, -14.5504)
  point P10 (17.0001, 14.3066)
  point P11 (37.0001, 14.3066)
  point P12 (37.0001, 14.3066)
  point P13 (17.0001, 43.1636)
  point P14 (37.0001, 43.1636)
  point P15 (37.0001, 43.1636)
  point P16 (17.0001, 72.0206)
  point P17 (37.0001, 72.0206)
  point P18 (37.0001, 72.0206)
  dimension "d217" = 23.734
  dimension "d218" = 16
  dimension "d219" = 23
  dimension "d220" = 14
  dimension "d221" = 23.734
  dimension "d222" = 16
  dimension "d223" = 23
  dimension "d224" = 14
  dimension "d225" = 23.734
  dimension "d226" = 16
  dimension "d227" = 23
  dimension "d228" = 14
  dimension "d229" = 23.734
  dimension "d230" = 16
  dimension "d231" = 23
  dimension "d232" = 14
  dimension "d233" = 23.734
  dimension "d234" = 16
  dimension "d235" = 23
  dimension "d236" = 14
  dimension "d237" = 23.734
  dimension "d238" = 16
  dimension "d239" = 23
  dimension "d240" = 14
  constraints: 328 end point, 72 midpoint, 24 parallel, 19 vertical, 13 perpendicular, 11 symmetric about line, 6 horizontal
  measures "d217" distance of L3.start L3.end
  measures "d218" distance of L4.end L3.end
  measures "d219" distance of L10.start L10.end
  measures "d220" distance of L11.end L10.end
  measures "d221" distance of L35.start L32.start
  measures "d222" distance of L32.end L32.start
  measures "d223" distance of L42.start L39.start
  measures "d224" distance of L39.end L39.start
  measures "d225" distance of L62.start L59.start
  measures "d226" distance of L59.end L59.start
  measures "d227" distance of L69.start L66.start
  measures "d228" distance of L66.end L66.start
  measures "d229" distance of L89.start L86.start
  measures "d230" distance of L86.end L86.start
  measures "d231" distance of L96.start L93.start
  measures "d232" distance of L93.end L93.start
  measures "d233" distance of L116.start L113.start
  measures "d234" distance of L113.end L113.start
  measures "d235" distance of L123.start L120.start
  measures "d236" distance of L120.end L120.start
  measures "d237" distance of L143.start L140.start
  measures "d238" distance of L140.end L140.start
  measures "d239" distance of L150.start L147.start
  measures "d240" distance of L147.end L147.start
extrude "Extrusión12" cut sketch "Boceto12" against normal blind 1.5 contours L146 L149 L148 L147 | L141 L140 L139 L145 L137 | L137 L145 L139 L142 L141 | L119 L122 L121 L120 | L114 L113 L112 L118 L110 | L110 L118 L112 L115 L114 | L92 L95 L94 L93 | L87 L86 L85 L91 L83 | L83 L91 L85 L88 L87 | L65 L68 L67 L66 | L60 L59 L58 L64 L56 | L56 L64 L58 L61 L60 | L38 L41 L40 L39 | L33 L32 L31 L37 L2 | L2 L37 L31 L34 L33 | L10 L13 L12 L11 | L5 L4 L3 L9 L0 | L0 L9 L3 L6 L5 | L17 L18 L19 L20 | L23 L24 L25 L26 | L44 L45 L49 L46 | L50 L51 L55 L52 | L71 L72 L76 L73 | L77 L78 L82 L79 | L98 L99 L103 L100 | L104 L105 L109 L106 | L125 L126 L130 L127 | L131 L132 L136 L133 | L152 L153 L157 L154 | L158 L159 L163 L160